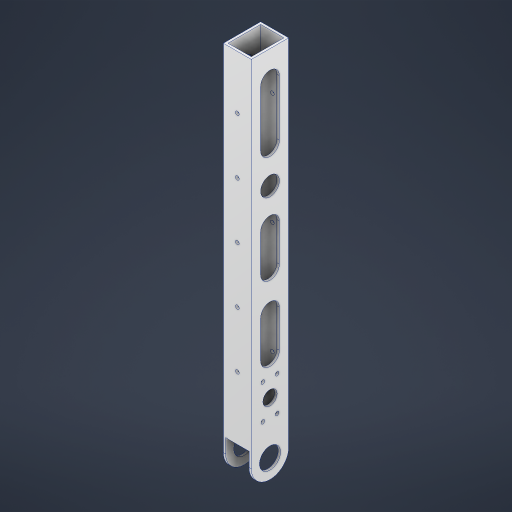
# Autodesk Inventor part: CLIM_002_ClimbPole
Saved by Autodesk Inventor 2024.2 (Build 282272000, 272)
## iProperties
Created: 2024-08-08
Part Number: CLIM_002_ClimbPole
Material: Aluminum 6061
Document SubType Name: Modeling
Designer: Bryan
Density: 2.7 g/cm^3
Appearance: Aluminum - Flat
Mass: 551.258 g
Surface Area: 1363.07 cm^2
Volume: 204.169 cm^3
Author: Bryan
Autodesk Inventor part; units mm, degrees
ref_plane "YZ Plane" through (0, 0, 0) normal (1, 0, 0) x (0, 1, 0)
ref_plane "XZ Plane" through (0, 0, 0) normal (0, 1, 0) x (-1, 0, 0)
ref_plane "XY Plane" through (0, 0, 0) normal (0, 0, 1) x (1, 0, 0)
sketch "Sketch1" plane through (0, 0, 0) normal (0, 1, 0) x (-1, 0, 0)
  line L0 (-19.05, -25.4) -> (19.05, -25.4)
  line L1 (19.05, -25.4) -> (19.05, 25.4)
  line L2 (19.05, 25.4) -> (-19.05, 25.4)
  line L3 (-19.05, 25.4) -> (-19.05, -25.4)
  line L4 (-19.05, -25.4) -> (19.05, 25.4) construction
  line L5 (19.05, -25.4) -> (-19.05, 25.4) construction
  line L6 (-15.875, 22.225) -> (15.875, 22.225)
  line L7 (15.875, 22.225) -> (15.875, -22.225)
  line L8 (15.875, -22.225) -> (-15.875, -22.225)
  line L9 (-15.875, -22.225) -> (-15.875, 22.225)
  point P0 (0, 0)
  dimension "d0" = 38.1
  dimension "d1" = 50.8
  dimension "d2" = 3.175
  constraints: 20 end point, 4 parallel, 2 midpoint, 2 perpendicular, 1 horizontal, 3 other
  measures "d0" distance of L2.end L1.end
  measures "d1" distance of L1.end L0.end
  measures "d2" distance between parallel lines of L2 L6
extrude "Extrusion1" add sketch "Sketch1" along normal blind 508
sketch "Sketch2" plane through (19.05, 0, 25.4) normal (1, 0, 0) x (0, 0, -1)
  line L0 (25.4, 469.9) -> (25.4, 393.7) construction
  line L1 (12.7, 469.9) -> (12.7, 393.7)
  line L2 (38.1, 393.7) -> (38.1, 469.9)
  arc A0 (38.1, 469.9) -> (12.7, 469.9) centre (25.4, 469.9) ccw
  arc A1 (12.7, 393.7) -> (38.1, 393.7) centre (25.4, 393.7) ccw
  line L3 (25.4, 298.45) -> (25.4, 146.05) construction
  line L4 (12.7, 298.45) -> (12.7, 146.05)
  line L5 (38.1, 146.05) -> (38.1, 298.45)
  arc A2 (38.1, 298.45) -> (12.7, 298.45) centre (25.4, 298.45) ccw
  arc A3 (12.7, 146.05) -> (38.1, 146.05) centre (25.4, 146.05) ccw
  line L6 (25.4, 114.3) -> (25.4, 38.1) construction
  line L7 (12.7, 114.3) -> (12.7, 38.1)
  line L8 (38.1, 38.1) -> (38.1, 114.3) construction
  arc A4 (38.1, 114.3) -> (12.7, 114.3) centre (25.4, 114.3) ccw
  arc A5 (12.7, 38.1) -> (38.1, 38.1) centre (25.4, 38.1) ccw construction
  line L9 (0, 0) -> (50.8, 0) projected
  line L10 (50.8, 0) -> (50.8, 508) projected
  line L11 (0, 508) -> (50.8, 508) projected
  line L12 (0, 0) -> (0, 508) projected
  line L13 (0, 0) -> (0, 508) projected
  circle A6 centre (25.4, 346.075) radius 12.7
  circle A7 centre (25.4, 25.4) radius 25.4
  circle A8 centre (25.4, 25.4) radius 14.2875
  circle A9 centre (25.4, 222.25) radius 12.7
  arc A10 (12.7, 247.65) -> (38.1, 247.65) centre (25.4, 247.65) ccw
  arc A11 (38.1, 196.85) -> (12.7, 196.85) centre (25.4, 196.85) ccw
  point P0 (25.4, 0)
  point P1 (25.4, 431.8)
  point P2 (25.4, 76.2)
  point P3 (25.4, 0)
  point P4 (25.4, 0)
  point P5 (0, 25.4)
  point P6 (50.8, 25.4)
  dimension "d5" = 25.4
  dimension "d6" = 25.4
  dimension "d7" = 25.4
  dimension "d8" = 508
  dimension "d9" = 76.2
  dimension "d10" = 152.4
  dimension "d11" = 76.2
  dimension "d15" = 25.4
  dimension "d16" = 161.925
  dimension "d18" = 38.1
  dimension "d19" = 38.1
  dimension "d35" = 28.575
  dimension "d49" = 298.45
  dimension "d52" = 25.4
  constraints: 24 end point, 21 tangent, 16 point on circle, 12 centre point, 8 point on line, 4 midpoint, 3 parallel, 2 coincident, 2 vertical alignment, 1 vertical
  measures "d5" diameter of A1
  measures "d6" diameter of A3
  measures "d7" diameter of A5
  measures "d8" distance of L9.end L10.end
  measures "d9" distance of L0.end L0.start
  measures "d10" distance of L3.start L3.end
  measures "d11" distance of L6.start L6.end
  measures "d15" diameter of A6
  measures "d16" distance from line of L11 A6.centre
  measures "d18" distance from line of L11 L0.start
  measures "d19" distance from line of L9 L6.end
  measures "d35" diameter of A8
  measures "d49" distance from line of L9 L3.start
  measures "d52" diameter of A9
extrude "Extrusion2" cut sketch "Sketch2" against normal blind 508 contours A0 L2 A1 L1 | A2 L5 A10 L4 | A11 L5 A3 L4 | L12 A7 L9 | A7 L10 L9 | A6 | A8
sketch "Sketch3" plane through (-19.05, 0, 25.4) normal (0, 0, 1) x (1, 0, 0)
  line L0 (19.05, 0) -> (19.05, 50.8) construction
  line L1 (19.05, 50.8) -> (19.05, 508) construction
  circle A0 centre (19.05, 53.975) radius 2.4892
  circle A1 centre (19.05, 130.175) radius 2.4892
  circle A2 centre (19.05, 206.375) radius 2.4892
  circle A3 centre (19.05, 282.575) radius 2.4892
  circle A4 centre (19.05, 358.775) radius 2.4892
  circle A5 centre (19.05, 434.975) radius 2.4892
  dimension "d20" = 50.8
  dimension "d21" = 457.2
  dimension "d22" = 4.9784
  dimension "d23" = 3.175
  dimension "d26" = 76.2
  constraints: 6 centre point, 4 end point, 3 vertical, 1 point on line, 10 other
  measures "d20" distance of L0.start L0.end
  measures "d21" distance of L0.end L1.end
  measures "d22" diameter of A0
  measures "d23" distance of L0.end A0.centre
  measures "d26" distance of A0.centre A1.centre
extrude "Extrusion3" cut sketch "Sketch3" against normal through all contours A1 | A2 | A3 | A4 | A5
sketch "Sketch5" plane through (-15.875, 508, 22.225) normal (1, 0, 0) x (0, 0, -1)
  circle A0 centre (22.225, -482.6) radius 14.2875 projected
  circle A1 centre (22.225, -482.6) radius 26.9875
  point P0 (22.225, -508)
  dimension "d36" = 53.975
  constraints: 1 centre point, 1 coincident
  measures "d36" diameter of A1
extrude "Extrusion5" cut sketch "Sketch5" along normal up to surface (31.75 mm away)
sketch "Sketch6" plane through (19.05, 508, 25.4) normal (1, 0, 0) x (0, 0, -1)
  circle A0 centre (25.4, -411.5562) radius 9.6012
  circle A1 centre (25.4, -411.5562) radius 25.4 construction
  line L0 (15.6798, -388.0897) -> (35.1202, -388.0897) construction
  line L1 (35.1202, -388.0897) -> (35.1202, -435.0227) construction
  line L2 (35.1202, -435.0227) -> (15.6798, -435.0227) construction
  line L3 (15.6798, -435.0227) -> (15.6798, -388.0897) construction
  arc A2 (0, -482.6) -> (50.8, -482.6) centre (25.4, -482.6) ccw projected
  circle A3 centre (15.6798, -388.0897) radius 2.4892
  circle A4 centre (1.9335, -401.836) radius 2.4892 construction
  circle A5 centre (1.9335, -421.2764) radius 2.4892 construction
  circle A6 centre (15.6798, -435.0227) radius 2.4892
  circle A7 centre (35.1202, -435.0227) radius 2.4892
  circle A8 centre (48.8665, -421.2764) radius 2.4892 construction
  circle A9 centre (48.8665, -401.836) radius 2.4892 construction
  circle A10 centre (35.1202, -388.0897) radius 2.4892
  point P0 (25.4, -508)
  point P1 (25.4, -508)
  dimension "d39" = 19.2024
  dimension "d40" = 50.8
  dimension "d41" = 4.9784
  dimension "d44" = 360
  dimension "d46" = 71.0438
  constraints: 10 centre point, 8 end point, 4 point on circle, 3 coincident, 2 parallel, 1 horizontal, 1 perpendicular, 1 vertical alignment, 17 other
  measures "d39" diameter of A0
  measures "d40" diameter of A1
  measures "d41" diameter of A3
  measures "d46" distance of A2.centre A0.centre
extrude "Extrusion6" cut sketch "Sketch6" against normal blind 25.4
sketch "Sketch8" plane through (-19.05, 508, -25.4) normal (-1, 0, 0) x (0, 0, 1)
  circle A0 centre (25.4, -411.5562) radius 9.6012 projected
  circle A1 centre (25.4, -411.5562) radius 15.875
  point P0 (25.4, -508)
  dimension "d53" = 31.75
  constraints: 1 centre point, 1 coincident
  measures "d53" diameter of A1
extrude "Extrusion7" cut sketch "Sketch8" against normal blind 25.4 contours A0 | A1
sketch "Sketch9" plane through (19.05, 508, -25.4) normal (0, 0, -1) x (-1, 0, 0)
  line L0 (34.925, -467.2907) -> (3.175, -467.2907) projected
  line L1 (3.175, -467.2907) -> (3.175, -473.4805) projected
  line L2 (34.925, -467.2907) -> (34.925, -473.4805) projected
  line L3 (3.175, -473.4805) -> (34.925, -473.4805) projected
  line L4 (3.175, -467.2907) -> (3.175, -463.4807)
  line L5 (3.175, -467.2907) -> (3.175, 0) projected
  line L6 (3.175, -463.4807) -> (34.925, -463.4807)
  line L7 (34.925, -467.2907) -> (34.925, 0) projected
  point P0 (19.05, -508)
  dimension "d64" = 3.81
  constraints: 4 end point, 2 point on line, 1 horizontal
  measures "d64" distance of L0.end L4.end
extrude "Extrusion8" cut sketch "Sketch9" against normal through all
sketch "Sketch10" plane through (19.05, 508, 25.4) normal (1, 0, 0) x (0, 0, -1)
  circle A0 centre (25.4, -482.6) radius 14.2875 projected
  circle A1 centre (25.4, -482.6) radius 22.225
  line L0 (50.8, -482.6) -> (50.8, 0) projected
  arc A2 (25.4, -504.825) -> (50.8, -479.425) centre (25.4, -479.425) ccw
  line L1 (0, -482.6) -> (0, 0) projected
  arc A3 (0, -479.425) -> (25.4, -504.825) centre (25.4, -479.425) ccw
  arc A4 (0, -482.6) -> (50.8, -482.6) centre (25.4, -482.6) ccw projected
  point P0 (25.4, -508)
  point P1 (25.4, -504.825)
  dimension "d58" = 44.45
  constraints: 6 point on circle, 4 tangent, 3 centre point, 2 coincident, 2 point on line, 1 vertical alignment
  measures "d58" diameter of A1
extrude "Extrusion9" [suppressed]
chamfer "Chamfer1" distance 3.175 angle 45 2 edges at (0, 44.5193, -22.225) (0, 44.5193, 22.225)
body "Solid1"
